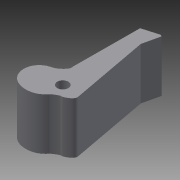
# Autodesk Inventor part: FelixOriginalHandle
Saved by Autodesk Inventor 2015 SP1 (Build 190203100, 203)
## iProperties
Created: 2014-12-14
Part Number: FelixOriginalHandle
Material: Generic
Document SubType Name: Modeling
Designer: Jack
Density: 1 g/cm^3
Appearance: Default
Author: Jack
Autodesk Inventor part; units mm, degrees
ref_plane "YZ Plane" through (0, 0, 0) normal (1, 0, 0) x (0, 1, 0)
ref_plane "XZ Plane" through (0, 0, 0) normal (0, 1, 0) x (-1, 0, 0)
ref_plane "XY Plane" through (0, 0, 0) normal (0, 0, 1) x (1, 0, 0)
sketch "Sketch1" plane through (0, 0, 0) normal (0, 0, 1) x (1, 0, 0)
  line L0 (0, 0) -> (86.2249, 0) construction
  line L1 (86.2249, 0) -> (86.2249, -43.5625) construction
  line L2 (86.2249, -43.5625) -> (0, -43.5625) construction
  line L3 (0, -43.5625) -> (0, 0) construction
  circle A0 centre (41.05, -33.8) radius 2
  line L4 (43.0565, -0.6221) -> (43.7124, -0.9832)
  line L5 (43.7124, -0.9832) -> (42.3228, -7.0446)
  line L6 (42.3228, -7.0446) -> (47.5119, -34.7478)
  line L7 (43.0565, -0.6221) -> (37.3078, -2.2779)
  line L8 (37.3078, -2.2779) -> (37.1832, -26.334)
  arc A1 (33.0926, -30.4146) -> (29.0233, -35.9297) centre (34.6218, -35.8017) ccw
  arc A2 (29.0233, -35.9297) -> (32.2264, -41.0137) centre (34.8718, -35.796) ccw
  arc A3 (32.2264, -41.0137) -> (37.836, -41.616) centre (35.8257, -33.9145) ccw
  arc A4 (37.836, -41.616) -> (41.5511, -39.09) centre (36.1433, -35.1314) ccw
  arc A5 (47.3778, -35.6783) -> (47.5119, -34.7478) centre (45.9681, -35.0003) ccw
  arc A6 (33.0926, -30.4146) -> (34.6145, -29.8918) centre (30.9901, -21.818) ccw
  arc A7 (36.9394, -27.7596) -> (37.1832, -26.334) centre (35.7821, -26.828) ccw
  arc A8 (34.6145, -29.8918) -> (36.9394, -27.7596) centre (31.5679, -24.2361) ccw
  arc A9 (43.8095, -37.6744) -> (41.5511, -39.09) centre (47.2093, -45.6075) ccw
  arc A10 (46.5697, -36.5667) -> (47.3778, -35.6783) centre (44.7183, -34.071) ccw
  arc A11 (44.8599, -37.5068) -> (46.5697, -36.5667) centre (42.2678, -30.7678) ccw
  arc A12 (44.3265, -37.5869) -> (44.8599, -37.5068) centre (44.4128, -36.3443) ccw
  arc A13 (44.3265, -37.5869) -> (43.8095, -37.6744) centre (44.2491, -38.7003) ccw
  dimension "d2" = 4
  dimension "d30" = 41.05
  dimension "d31" = 33.8
  dimension "d35" = 86.225
  constraints: 26 point on circle, 14 centre point, 12 end point, 7 tangent, 1 coincident, 20 other
  measures "d2" diameter of A0
  measures "d30" horizontal distance of point (0, 0) A0.centre
  measures "d31" vertical distance of L0.start A0.centre
  measures "d35" distance of L0.start L0.end
extrude "Extrusion1" add sketch "Sketch1" along normal blind 18.5
body "Solid1"
